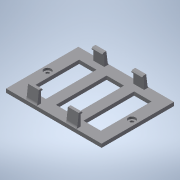
# Autodesk Inventor part: breadboard clip - edit
Saved by Autodesk Inventor 2020 (Build 240168000, 168)
## iProperties
Created: 2017-08-14
Part Number: breadboard clip - edit
Material: Generic
Document SubType Name: Modeling
Designer: kteo17
Density: 1 g/cm^3
Appearance: Default
Author: kteo17
## iProperties of the stored document _3DPrint.ipt
Created: 2019-06-03
Part Number: _3DPrint
Material: Generic
Document SubType Name: Modeling
Designer: cruss
Density: 1 g/cm^3
Appearance: Default
Author: cruss
Autodesk Inventor part; units mm, degrees
ref_plane "YZ Plane" through (0, 0, 0) normal (1, 0, 0) x (0, 1, 0)
ref_plane "XZ Plane" through (0, 0, 0) normal (0, 1, 0) x (-1, 0, 0)
ref_plane "XY Plane" through (0, 0, 0) normal (0, 0, 1) x (1, 0, 0)
sketch "Sketch1" plane through (0, 0, 0) normal (0, 1, 0) x (-1, 0, 0)
  line L0 (0, 0) -> (83.82, 0)
  line L1 (83.82, 0) -> (83.82, 63.5)
  line L2 (83.82, 63.5) -> (0, 63.5)
  line L3 (0, 63.5) -> (0, 0)
  line L4 (73.66, 53.975) -> (58.42, 53.975)
  line L5 (58.42, 53.975) -> (58.42, 9.525)
  line L6 (58.42, 9.525) -> (73.66, 9.525)
  line L7 (73.66, 9.525) -> (73.66, 53.975)
  line L8 (49.53, 53.975) -> (34.29, 53.975)
  line L9 (34.29, 53.975) -> (34.29, 9.525)
  line L10 (34.29, 9.525) -> (49.53, 9.525)
  line L11 (49.53, 9.525) -> (49.53, 53.975)
  line L12 (25.4, 53.975) -> (10.16, 53.975)
  line L13 (10.16, 53.975) -> (10.16, 9.525)
  line L14 (10.16, 9.525) -> (25.4, 9.525)
  line L15 (25.4, 9.525) -> (25.4, 53.975)
  dimension "d0" = 83.82
  dimension "d1" = 63.5
  dimension "d41" = 10.16
  dimension "d42" = 8.89
  dimension "d43" = 8.89
  dimension "d44" = 15.24
  dimension "d45" = 15.24
  dimension "d46" = 15.24
  constraints: 32 end point, 8 parallel, 4 horizontal, 4 perpendicular
  measures "d0" distance of L2.end L1.end
  measures "d1" distance of L1.end L0.end
  measures "d41" distance between parallel lines of L7 L1
  measures "d42" distance between parallel lines of L11 L5
  measures "d43" distance between parallel lines of L15 L9
  measures "d44" distance of L5.end L6.end
  measures "d45" distance of L9.end L10.end
  measures "d46" distance of L13.end L14.end
extrude "Extrusion1" add sketch "Sketch1" along normal blind 3.175
sketch "Sketch4" plane through (0, 3.175, 0) normal (0, 1, 0) x (1, 0, 0)
  line L0 (-83.82, -63.5) -> (0, -63.5) projected
  line L1 (0, 0) -> (-83.82, 0) projected
  line L2 (-66.675, 0) -> (-57.15, 0)
  line L3 (-57.15, 0) -> (-57.15, -3.9624)
  line L4 (-57.15, -3.9624) -> (-66.675, -3.9624)
  line L5 (-66.675, -3.9624) -> (-66.675, 0)
  line L6 (-31.75, 0) -> (-22.225, 0)
  line L7 (-22.225, 0) -> (-22.225, -3.9624)
  line L8 (-22.225, -3.9624) -> (-31.75, -3.9624)
  line L9 (-31.75, -3.9624) -> (-31.75, 0)
  line L10 (-66.675, -63.5) -> (-57.15, -63.5)
  line L11 (-57.15, -63.5) -> (-57.15, -59.5376)
  line L12 (-57.15, -59.5376) -> (-66.675, -59.5376)
  line L13 (-66.675, -59.5376) -> (-66.675, -63.5)
  line L14 (-31.75, -63.5) -> (-22.225, -63.5)
  line L15 (-22.225, -63.5) -> (-22.225, -59.5376)
  line L16 (-22.225, -59.5376) -> (-31.75, -59.5376)
  line L17 (-31.75, -59.5376) -> (-31.75, -63.5)
  constraints: 32 end point, 8 parallel, 4 horizontal, 4 perpendicular, 4 point on line
extrude "Extrusion4" add sketch "Sketch4" along normal blind 11.1252
sketch "Sketch5" plane through (-22.225, 3.175, 63.5) normal (1, 0, 0) x (0, 0, -1)
  line L0 (3.9624, 0) -> (0, 0) projected
  line L1 (3.9624, 0) -> (3.9624, 11.1252) projected
  line L2 (0, 11.1252) -> (3.9624, 11.1252) projected
  line L3 (0, 0) -> (0, 11.1252) projected
  line L4 (3.9624, 12.7) -> (2.1844, 12.7)
  line L5 (3.9624, -0.6232) -> (0.7874, -0.6232)
  line L6 (2.1844, 11.1252) -> (0.7874, 0)
  line L7 (0.7874, 0) -> (0, 0)
  line L8 (0, 0) -> (0, 11.1252)
  line L9 (0, 11.1252) -> (2.1844, 11.1252)
  line L10 (59.5376, 0) -> (63.5, 0)
  line L11 (59.5376, 0) -> (59.5376, 11.1252)
  line L12 (63.5, 11.1252) -> (59.5376, 11.1252)
  line L13 (63.5, 0) -> (63.5, 11.1252)
  line L14 (59.5376, 12.7) -> (61.3156, 12.7)
  line L15 (59.5376, -0.6232) -> (62.7126, -0.6232)
  line L16 (61.3156, 11.1252) -> (62.7126, 0)
  line L17 (62.7126, 0) -> (63.5, 0)
  line L18 (63.5, 0) -> (63.5, 11.1252)
  line L19 (63.5, 11.1252) -> (61.3156, 11.1252)
  point P0 (63.5, -3.175)
  dimension "d17" = 1.778
  dimension "d18" = 3.175
  constraints: 32 end point, 6 point on line, 3 collinear, 1 parallel, 1 perpendicular
  measures "d17" distance of L4.start L4.end
  measures "d18" distance of L5.start L5.end
extrude "Extrusion5" cut sketch "Sketch5" against normal blind 44.45 contours L0 L3 L2 L6 | L16 L12 L13 L10
fillet "Fillet1" radius 3.175 4 edges at (-61.9125, 3.175, 62.7126) (-26.9875, 3.175, 62.7126) (-26.9875, 3.175, 0.7874) (-61.9125, 3.175, 0.7874)
sketch "Sketch6" plane through (0, 14.3002, 0) normal (0, 1, 0) x (1, 0, 0)
  line L0 (-22.225, -59.5376) -> (-31.75, -59.5376) projected
  line L1 (-31.75, -59.5376) -> (-22.225, -59.5376)
  line L2 (-22.225, -59.5376) -> (-22.225, -57.912)
  line L3 (-22.225, -57.912) -> (-31.75, -57.912)
  line L4 (-31.75, -57.912) -> (-31.75, -59.5376)
  line L5 (-57.15, -59.5376) -> (-66.675, -59.5376)
  line L6 (-66.675, -59.5376) -> (-66.675, -57.912)
  line L7 (-66.675, -57.912) -> (-57.15, -57.912)
  line L8 (-57.15, -57.912) -> (-57.15, -59.5376)
  line L9 (-31.75, -2.1844) -> (-22.225, -2.1844)
  line L10 (-22.225, -2.1844) -> (-22.225, -3.9624)
  line L11 (-22.225, -3.9624) -> (-31.75, -3.9624)
  line L12 (-31.75, -3.9624) -> (-31.75, -2.1844)
  line L13 (-31.75, -3.9624) -> (-22.225, -3.9624)
  line L14 (-22.225, -3.9624) -> (-22.225, -5.588)
  line L15 (-22.225, -5.588) -> (-31.75, -5.588)
  line L16 (-31.75, -5.588) -> (-31.75, -3.9624)
  line L17 (-57.15, -3.9624) -> (-66.675, -3.9624)
  line L18 (-66.675, -3.9624) -> (-66.675, -5.588)
  line L19 (-66.675, -5.588) -> (-57.15, -5.588)
  line L20 (-57.15, -5.588) -> (-57.15, -3.9624)
  line L21 (-66.675, -3.9624) -> (-57.15, -3.9624) projected
  point P0 (0, 0)
  dimension "d50" = 1.6256
  dimension "d51" = 1.6256
  dimension "d52" = 1.6256
  dimension "d53" = 1.6256
  dimension "d54" = 0
  constraints: 40 end point, 4 parallel, 2 horizontal, 2 perpendicular, 2 point on line
  measures "d50" distance of L7.end L5.start
  measures "d51" distance of L1.end L2.end
  measures "d52" distance of L19.end L17.start
  measures "d53" distance of L15.end L13.start
  measures "d54" distance between parallel lines of L21 L17
extrude "Extrusion6" add sketch "Sketch6" against normal blind 1.6002 contours L0 L4 L3 L2 | L5 L6 L7 L8 | L11 L14 L15 L16 | L20 L19 L18 L17
sketch "Sketch7" plane through (-22.225, 3.175, 63.5) normal (1, 0, 0) x (0, 0, -1)
  line L0 (5.588, 11.1252) -> (5.588, 9.525) projected
  line L1 (2.1844, 11.1252) -> (5.588, 11.1252) projected
  line L2 (4.5974, 11.1252) -> (5.588, 9.525)
  line L3 (4.5974, 11.1252) -> (5.588, 11.1252)
  line L4 (5.588, 9.525) -> (5.588, 11.1252)
  line L5 (61.3156, 11.1252) -> (62.4649, 1.9722)
  arc A0 (62.4649, 1.9722) -> (63.5, 0) centre (65.6152, 2.3678) ccw
  line L6 (59.5376, 0) -> (63.5, 0)
  line L7 (59.5376, 0) -> (59.5376, 9.525)
  line L8 (57.15, 9.525) -> (59.5376, 9.525)
  line L9 (57.15, 11.1252) -> (57.15, 9.525)
  line L10 (61.3156, 11.1252) -> (57.15, 11.1252)
  line L11 (58.9026, 11.1252) -> (57.15, 9.525)
  line L12 (58.9026, 11.1252) -> (57.15, 11.1252)
  line L13 (57.15, 9.525) -> (57.15, 11.1252)
  point P0 (63.5, -3.175)
  constraints: 24 end point, 2 point on circle, 2 point on line, 1 centre point, 1 collinear, 1 perpendicular
extrude "Extrusion7" cut sketch "Sketch7" against normal blind 44.45 contours L0 L2 L1 | L11 L9 L10
sketch "Sketch8" plane through (0, 3.175, 0) normal (0, 1, 0) x (1, 0, 0)
  circle A0 centre (-79.0956, -31.75) radius 3.175
  circle A1 centre (-5.08, -31.75) radius 3.1695
  line L0 (0, -63.5) -> (0, 0) projected
  line L1 (-66.675, 0) -> (-83.82, 0) projected
  line L2 (0, 0) -> (-22.225, 0) projected
  dimension "d29" = 74.0156
  dimension "d47" = 5.08
  dimension "d48" = 31.75
  dimension "d49" = 31.75
  constraints: 2 centre point
  measures "d29" distance of A1.centre A0.centre
  measures "d47" distance from line of A1.centre L0
  measures "d48" distance from line of L1 A0.centre
  measures "d49" distance from line of L2 A1.centre
extrude "Extrusion8" cut sketch "Sketch8" against normal blind 1.905
sketch "Sketch9" plane through (0, 3.175, 0) normal (0, 1, 0) x (1, 0, 0)
  circle A0 centre (-5.08, -31.75) radius 3.1695 projected
  circle A1 centre (-79.0956, -31.75) radius 3.175 projected
  circle A2 centre (-79.0956, -31.75) radius 1.5875
  circle A3 centre (-5.08, -31.75) radius 1.5875
  constraints: 2 centre point, 2 coincident
extrude "Extrusion9" cut sketch "Sketch9" against normal blind 3.175 contours A2 | A3
sketch "Sketch12" plane through (0, 12.7, 0) normal (0, -1, 0) x (1, 0, 0)
  line L0 (-22.225, 3.9624) -> (-22.225, 5.588) projected
  line L1 (-22.225, 5.588) -> (-31.75, 5.588) projected
  line L2 (-22.225, 3.9624) -> (-31.75, 3.9624)
  line L3 (-31.75, 3.9624) -> (-31.75, 5.588)
  line L4 (-31.75, 5.588) -> (-22.225, 5.588)
  line L5 (-22.225, 5.588) -> (-22.225, 3.9624)
  line L6 (-57.15, 3.9624) -> (-66.675, 3.9624) projected
  line L7 (-57.15, 5.588) -> (-66.675, 5.588) projected
  line L8 (-57.15, 3.9624) -> (-66.675, 3.9624)
  line L9 (-66.675, 3.9624) -> (-66.675, 5.588)
  line L10 (-66.675, 5.588) -> (-57.15, 5.588)
  line L11 (-57.15, 5.588) -> (-57.15, 3.9624)
  line L12 (-66.675, 57.912) -> (-57.15, 57.912) projected
  line L13 (-57.15, 59.5376) -> (-66.675, 59.5376)
  line L14 (-66.675, 59.5376) -> (-66.675, 57.912)
  line L15 (-66.675, 57.912) -> (-57.15, 57.912)
  line L16 (-57.15, 57.912) -> (-57.15, 59.5376)
  line L17 (-31.75, 57.912) -> (-22.225, 57.912) projected
  line L18 (-31.75, 59.5376) -> (-22.225, 59.5376) projected
  line L19 (-22.225, 57.912) -> (-31.75, 57.912)
  line L20 (-31.75, 57.912) -> (-31.75, 59.5376)
  line L21 (-31.75, 59.5376) -> (-22.225, 59.5376)
  line L22 (-22.225, 59.5376) -> (-22.225, 57.912)
  point P0 (0, 0)
  constraints: 32 end point, 8 parallel, 4 horizontal, 4 perpendicular
equation "\"d43\" = d42"
equation "\"d45\" = d44"
equation "\"d46\" = d44"
equation "\"d51\" = d50"
equation "\"d52\" = d50"
equation "\"d53\" = d50"
body "Solid1"
